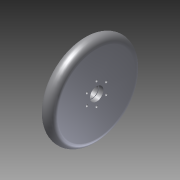
# Autodesk Inventor part: pneumatic 8'' wheel sketchy quality
Saved by Autodesk Inventor 2011 SP1 (Build 150282100, 282)
## iProperties
Created: 2013-01-18
Part Number: pneumatic 8'' wheel sketchy quality
Document SubType Name: Modeling
Designer: wes
Density: 1 g/cm^3
Author: wes
Autodesk Inventor part; units mm, degrees
ref_plane "YZ Plane" through (0, 0, 0) normal (1, 0, 0) x (0, 1, 0)
ref_plane "XZ Plane" through (0, 0, 0) normal (0, 1, 0) x (-1, 0, 0)
ref_plane "XY Plane" through (0, 0, 0) normal (0, 0, 1) x (1, 0, 0)
sketch "Sketch1" plane through (0, 0, 0) normal (0, 0, 1) x (1, 0, 0)
  line L0 (-17.6048, 17.9341) -> (10.9702, 17.9341)
  line L1 (10.9702, 17.9341) -> (10.9702, -64.9334)
  line L2 (10.9702, -64.9334) -> (-17.6048, -64.9334)
  line L3 (-17.6048, -64.9334) -> (-17.6048, 17.9341)
  circle A0 centre (-3.3173, 17.9341) radius 14.2875
  point P0 (0, 0)
  dimension "d0" = 28.575
  dimension "d1" = 82.8675
  constraints: 8 end point, 2 parallel, 1 horizontal, 1 horizontal alignment, 1 midpoint, 1 perpendicular, 2 other
  measures "d0" distance between parallel lines of L1 L3
  measures "d1" distance from line of L2 point (-3.317, 17.934)
revolve "Revolution1" add sketch "Sketch1" angle 360 about axis through (10.9702, -64.9334, 0) along (-1, 0, 0)
sketch "Sketch2" plane through (10.9702, -64.9334, 0) normal (1, 0, 0) x (0, 0, -1)
  circle A0 centre (0, 0) radius 82.8675 projected
  circle A1 centre (0, 0) radius 23.8125
  circle A2 centre (0, 0) radius 12.7
  line L0 (0, 0) -> (0, 42.8884)
  line L1 (37.1175, 21.4298) -> (0, 0)
  line L2 (0, 0) -> (31.3254, -18.0857)
  line L3 (31.3254, -18.0857) -> (0, 0)
  line L4 (0, 0) -> (0, -34.1508)
  line L5 (0, -34.1508) -> (0, 0)
  line L6 (0, 0) -> (-30.532, -17.6277)
  line L7 (-30.532, -17.6277) -> (0, 0)
  line L8 (0, 0) -> (-29.5082, 17.0365)
  circle A3 centre (0, 0) radius 14.2875
  point P0 (0, 64.9334)
  point P1 (0, 23.8125)
  point P2 (20.6222, 11.9063)
  point P3 (20.6222, -11.9062)
  point P4 (0, -23.8125)
  point P5 (-20.6222, -11.9063)
  point P6 (-20.6222, 11.9062)
  dimension "d3" = 47.625
  dimension "d4" = 25.4
  dimension "d5" = 60
  dimension "d6" = 60
  dimension "d7" = 60
  dimension "d8" = 60
  dimension "d16" = 28.575
  constraints: 18 end point, 6 point on circle, 5 point on line, 4 collinear, 3 centre point, 3 coincident, 1 vertical
  measures "d3" diameter of A1
  measures "d4" diameter of A2
  measures "d5" angle of L1 L0
  measures "d6" angle of L2 L1
  measures "d7" angle of L4 L6
  measures "d8" angle of L6 L8
  measures "d16" diameter of A3
hole "Hole1" at (10.9702, -41.1209, 0) at (10.9702, -53.0271, -20.6222) at (10.9702, -76.8396, -20.6222) at (10.9702, -88.7459, 0) at (10.9702, -76.8396, 20.6222) at (10.9702, -53.0271, 20.6222) direction (-1, 0, 0) diameter 5.08 depth 50.8 tip angle 118
extrude "Extrusion1" cut sketch "Sketch2" against normal blind 50.8 contours L1 L0 A2 | A2 L2 L1 | A2 L4 L2 | L0 L8 A2 | L4 A2 L6 | L6 A2 L8
extrude "Extrusion2" cut sketch "Sketch2" against normal blind 9.525 contours A3 L2 A2 L1 | L1 A2 L0 A3 | A3 L4 A2 L2 | L0 A2 L8 A3 | A3 L6 A2 L4 | L8 A2 L6 A3
sketch "Sketch3" plane through (-17.6048, -64.9334, 0) normal (-1, 0, 0) x (0, 0, 1)
  circle A0 centre (0, 0) radius 12.7 projected
  circle A1 centre (0, 0) radius 82.8675 projected
  circle A2 centre (0, 0) radius 14.2875
  point P0 (0, 64.9334)
  dimension "d21" = 28.575
  constraints: 1 centre point, 1 coincident
  measures "d21" diameter of A2
extrude "Extrusion3" cut sketch "Sketch3" against normal blind 9.525 contours A2
body "Solid1"
